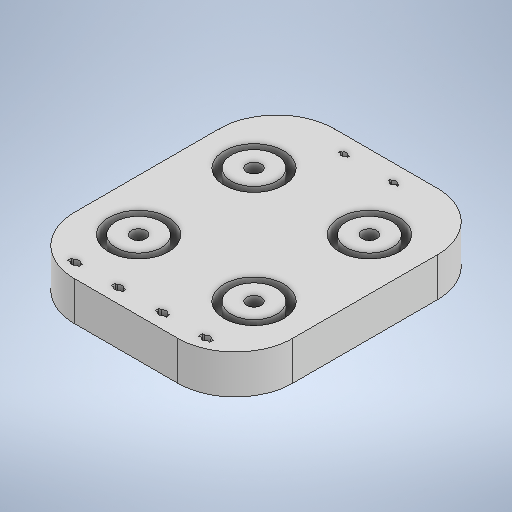
# Autodesk Inventor part: BlenderCase
Saved by Autodesk Inventor 2025 (Build 290162000, 162)
## iProperties
Created: 2025-02-08
Part Number: BlenderCase
Material: Generic
Document SubType Name: Modeling
Designer: ethan
Density: 1 g/cm^3
Appearance: Default
Author: ethan
Autodesk Inventor part; units mm, degrees
ref_plane "YZ Plane" through (0, 0, 0) normal (1, 0, 0) x (0, 1, 0)
ref_plane "XZ Plane" through (0, 0, 0) normal (0, 1, 0) x (-1, 0, 0)
ref_plane "XY Plane" through (0, 0, 0) normal (0, 0, 1) x (1, 0, 0)
sketch "Sketch1" plane through (0, 0, 0) normal (0, 1, 0) x (-1, 0, 0)
  circle A0 centre (0, 0) radius 26.1938
  circle A1 centre (0, 0) radius 19.8438
  circle A2 centre (0, 0) radius 32.5438
  dimension "d0" = 52.3875
  dimension "d1" = 6.35
  dimension "d2" = 6.35
  constraints: 3 centre point, 1 coincident
  measures "d0" diameter of A0
  measures "d1" radial gap between concentric circles of A0 A1
  measures "d2" radial gap between concentric circles of A0 A2
extrude "Extrusion1" add sketch "Sketch1" along normal blind 31.75
sketch "Sketch2" plane through (0, 31.75, 0) normal (0, 1, 0) x (1, 0, 0)
  circle A0 centre (0, 0) radius 6.35
  dimension "d5" = 12.7
  constraints: 1 centre point, 1 coincident
  measures "d5" diameter of A0
extrude "Extrusion2" cut sketch "Sketch2" against normal blind 31.75
sketch "Sketch3" plane through (0, 31.75, 0) normal (0, 1, 0) x (1, 0, 0)
  circle A0 centre (0, 0) radius 32.5438 construction
  circle A1 centre (0, 0) radius 32.5438 construction
  circle A2 centre (0, 0) radius 26.1938 construction
  circle A3 centre (0, 0) radius 26.1938 construction
  circle A4 centre (0, 0) radius 19.8438 construction
  circle A5 centre (0, 0) radius 19.8438 construction
  circle A6 centre (0, 0) radius 6.35 construction
  circle A7 centre (0, 0) radius 6.35 construction
  circle A8 centre (0, 0) radius 32.5438 construction
  circle A9 centre (0, 0) radius 26.1938 construction
  circle A10 centre (0, 0) radius 32.5438 construction
  circle A11 centre (0, 0) radius 26.1938 construction
  circle A12 centre (0, 0) radius 32.5438 construction
  circle A13 centre (0, 0) radius 32.5438 construction
  circle A14 centre (0, 0) radius 26.1938 construction
  circle A15 centre (0, 0) radius 26.1938 construction
  circle A16 centre (0, 0) radius 6.35 construction
  circle A17 centre (0, 0) radius 19.8438 construction
  circle A18 centre (0, 0) radius 6.35 construction
  circle A19 centre (0, 0) radius 19.8438 construction
  circle A20 centre (0, 0) radius 19.8438 construction
  circle A21 centre (0, 0) radius 19.8438 construction
  circle A22 centre (0, 0) radius 6.35 construction
  circle A23 centre (0, 0) radius 6.35 construction
  line L0 (0, 0) -> (101.6, 0) construction
  line L1 (101.6, 0) -> (101.6, -101.6) construction
  circle A24 centre (0, 0) radius 6.35
  circle A25 centre (0, 0) radius 19.8438
  circle A26 centre (0, 0) radius 26.1938
  circle A27 centre (0, 0) radius 32.5438
  circle A28 centre (101.6, 0) radius 19.8438
  circle A29 centre (101.6, 0) radius 26.1938
  circle A30 centre (101.6, 0) radius 6.35
  circle A31 centre (101.6, 0) radius 32.5438
  circle A32 centre (0, -101.6) radius 19.8438
  circle A33 centre (0, -101.6) radius 26.1938
  circle A34 centre (0, -101.6) radius 6.35
  circle A35 centre (0, -101.6) radius 32.5438
  circle A36 centre (101.6, -101.6) radius 19.8438
  circle A37 centre (101.6, -101.6) radius 26.1938
  circle A38 centre (101.6, -101.6) radius 6.35
  circle A39 centre (101.6, -101.6) radius 32.5438
  line L2 (0, 0) -> (50.8, 87.9882) construction
  line L3 (50.8, 87.9882) -> (101.6, 0) construction
  line L4 (16.2719, 28.1837) -> (28.9719, 50.1808) construction
  line L5 (28.9719, 50.1808) -> (72.6281, 50.1808) construction
  circle A40 centre (28.9719, 50.1808) radius 2.3812
  circle A41 centre (72.6281, 50.1808) radius 2.3813
  line L6 (25.0031, 49.387) -> (32.9406, 49.387)
  line L7 (32.9406, 49.387) -> (32.9406, 50.9745)
  line L8 (32.9406, 50.9745) -> (25.0031, 50.9745)
  line L9 (25.0031, 50.9745) -> (25.0031, 49.387)
  line L10 (25.0031, 49.387) -> (32.9406, 50.9745) construction
  line L11 (32.9406, 49.387) -> (25.0031, 50.9745) construction
  line L12 (68.6594, 49.387) -> (76.5969, 49.387)
  line L13 (76.5969, 49.387) -> (76.5969, 50.9745)
  line L14 (76.5969, 50.9745) -> (68.6594, 50.9745)
  line L15 (68.6594, 50.9745) -> (68.6594, 49.387)
  line L16 (68.6594, 49.387) -> (76.5969, 50.9745) construction
  line L17 (76.5969, 49.387) -> (68.6594, 50.9745) construction
  line L18 (28.9719, 52.562) -> (28.9719, 65.262) construction
  line L19 (-107.0093, 65.262) -> (-107.0093, -188.738) construction
  line L20 (-32.5438, -101.6) -> (-45.2437, -101.6) construction
  line L21 (134.1437, -101.6) -> (146.8437, -101.6) construction
  line L22 (-45.2437, -188.738) -> (146.8438, -188.738) construction
  line L23 (-45.2437, -188.738) -> (-45.2437, -163.338) construction
  line L24 (-45.2437, 65.262) -> (96.0437, 65.262) construction
  line L25 (146.8438, 65.262) -> (146.8438, -112.538) construction
  line L26 (96.0437, -163.338) -> (5.5563, -163.338) construction
  line L27 (-45.2437, -112.538) -> (-45.2437, 65.262) construction
  line L28 (-45.2437, -163.338) -> (-6.8237, -163.338) construction
  line L29 (-6.8237, -163.338) -> (-6.8237, -150.638) construction
  line L30 (-6.8237, -163.338) -> (31.5963, -163.338) construction
  line L31 (31.5963, -163.338) -> (70.0164, -163.338) construction
  line L32 (70.0164, -163.338) -> (108.4364, -163.338) construction
  line L33 (108.4364, -163.338) -> (146.8438, -163.338) construction
  circle A42 centre (-6.8237, -150.638) radius 3.175 construction
  circle A43 centre (31.5963, -150.638) radius 3.175 construction
  circle A44 centre (70.0164, -150.638) radius 3.175 construction
  circle A45 centre (108.4364, -150.638) radius 3.175 construction
  circle A46 centre (-6.8237, -150.638) radius 3.175
  circle A47 centre (31.5963, -150.638) radius 3.175
  circle A48 centre (70.0164, -150.638) radius 3.175
  circle A49 centre (108.4364, -150.638) radius 3.175
  line L34 (-11.5862, -152.2255) -> (-2.0612, -152.2255)
  line L35 (-2.0612, -152.2255) -> (-2.0612, -149.0505)
  line L36 (-2.0612, -149.0505) -> (-11.5862, -149.0505)
  line L37 (-11.5862, -149.0505) -> (-11.5862, -152.2255)
  line L38 (-11.5862, -152.2255) -> (-2.0612, -149.0505) construction
  line L39 (-2.0612, -152.2255) -> (-11.5862, -149.0505) construction
  line L40 (26.8338, -152.2255) -> (36.3588, -152.2255)
  line L41 (36.3588, -152.2255) -> (36.3588, -149.0505)
  line L42 (36.3588, -149.0505) -> (26.8338, -149.0505)
  line L43 (26.8338, -149.0505) -> (26.8338, -152.2255)
  line L44 (26.8338, -152.2255) -> (36.3588, -149.0505) construction
  line L45 (36.3588, -152.2255) -> (26.8338, -149.0505) construction
  line L46 (65.2539, -152.2255) -> (74.7789, -152.2255)
  line L47 (74.7789, -152.2255) -> (74.7789, -149.0505)
  line L48 (74.7789, -149.0505) -> (65.2539, -149.0505)
  line L49 (65.2539, -149.0505) -> (65.2539, -152.2255)
  line L50 (65.2539, -152.2255) -> (74.7789, -149.0505) construction
  line L51 (74.7789, -152.2255) -> (65.2539, -149.0505) construction
  line L52 (103.6739, -152.2255) -> (113.1989, -152.2255)
  line L53 (113.1989, -152.2255) -> (113.1989, -149.0505)
  line L54 (113.1989, -149.0505) -> (103.6739, -149.0505)
  line L55 (103.6739, -149.0505) -> (103.6739, -152.2255)
  line L56 (103.6739, -152.2255) -> (113.1989, -149.0505) construction
  line L57 (113.1989, -152.2255) -> (103.6739, -149.0505) construction
  line L58 (-45.2437, -163.338) -> (146.8438, -163.338)
  line L59 (146.8438, -163.338) -> (146.8438, 14.462)
  line L60 (146.8438, 65.262) -> (5.5563, 65.262)
  line L61 (-45.2437, 14.462) -> (-45.2437, -163.338)
  arc A50 (5.5563, 65.262) -> (-45.2437, 14.462) centre (5.5563, 14.462) ccw
  arc A51 (146.8438, 14.462) -> (96.0437, 65.262) centre (96.0438, 14.462) ccw
  arc A52 (96.0437, -163.338) -> (146.8438, -112.538) centre (96.0438, -112.538) ccw
  arc A53 (-45.2437, -112.538) -> (5.5563, -163.338) centre (5.5563, -112.538) ccw
  point P0 (31.2169, 49.387)
  point P1 (26.7268, 49.387)
  point P2 (26.7268, 50.9745)
  point P3 (31.2169, 50.9745)
  point P4 (74.8732, 49.387)
  point P5 (70.3831, 49.387)
  point P6 (70.3831, 50.9745)
  point P7 (74.8732, 50.9745)
  point P8 (-4.0741, -152.2255)
  point P9 (-9.5733, -152.2255)
  point P10 (-9.5733, -149.0505)
  point P11 (-4.0741, -149.0505)
  point P12 (34.346, -152.2255)
  point P13 (28.8467, -152.2255)
  point P14 (28.8467, -149.0505)
  point P15 (34.346, -149.0505)
  point P16 (72.766, -152.2255)
  point P17 (67.2667, -152.2255)
  point P18 (67.2667, -149.0505)
  point P19 (72.766, -149.0505)
  point P20 (111.186, -152.2255)
  point P21 (105.6868, -152.2255)
  point P22 (105.6868, -149.0505)
  point P23 (111.186, -149.0505)
  dimension "d20" = 4.7625
  dimension "d8" = 101.6
  dimension "d9" = 101.6
  dimension "d12" = 101.6
  dimension "d15" = 101.6
  dimension "d18" = 101.6
  dimension "d19" = 25.4
  dimension "d21" = 4.7625
  dimension "d22" = 7.9375
  dimension "d23" = 1.5875
  dimension "d24" = 7.9375
  dimension "d25" = 1.5875
  dimension "d26" = 12.7
  dimension "d27" = 254
  dimension "d28" = 12.7
  dimension "d29" = 12.7
  dimension "d30" = 25.4
  dimension "d31" = 38.42
  dimension "d32" = 12.7
  dimension "d33" = 38.42
  dimension "d34" = 38.42
  dimension "d35" = 38.42
  dimension "d36" = 6.35
  dimension "d37" = 6.35
  dimension "d38" = 6.35
  dimension "d39" = 6.35
  dimension "d40" = 9.525
  dimension "d41" = 3.175
  dimension "d42" = 9.525
  dimension "d43" = 3.175
  dimension "d44" = 9.525
  dimension "d45" = 3.175
  dimension "d46" = 9.525
  dimension "d47" = 3.175
  dimension "d48" = 50.8
  constraints: 124 end point, 26 centre point, 23 coincident, 16 parallel, 13 point on line, 12 midpoint, 11 perpendicular, 10 horizontal, 8 equal radius, 8 point on circle, 8 tangent, 6 vertical, 2 horizontal alignment, 2 line through centre, 1 collinear, 106 other
  measures "d8" distance of L0.start L0.end
  measures "d9" distance of L0.end L1.end
  measures "d12" distance of A25.centre A28.centre
  measures "d15" distance of A25.centre A32.centre
  measures "d18" distance of L2.start L2.end
  measures "d19" distance of L4.start L4.end
  measures "d21" diameter of A41
  measures "d22" distance of L6.start L6.end
  measures "d23" distance of L7.end L6.end
  measures "d24" distance of L12.start L12.end
  measures "d25" distance of L13.end L12.end
  measures "d26" distance of L18.start L18.end
  measures "d27" distance of L19.start L19.end
  measures "d28" distance of L20.start L20.end
  measures "d29" distance of L21.start L21.end
  measures "d30" distance of L22.start L23.end
  measures "d31" distance of L28.start L28.end
  measures "d32" distance of L28.end L29.end
  measures "d33" distance of L28.end L30.end
  measures "d34" distance of L30.end L31.end
  measures "d35" distance of L31.end L32.end
  measures "d36" diameter of A42
  measures "d37" diameter of A43
  measures "d38" diameter of A44
  measures "d39" diameter of A45
  measures "d40" distance of L34.start L34.end
  measures "d41" distance of L35.end L34.end
  measures "d42" distance of L40.start L40.end
  measures "d43" distance of L41.end L40.end
  measures "d44" distance of L46.start L46.end
  measures "d45" distance of L47.end L46.end
  measures "d46" distance of L52.start L52.end
  measures "d47" distance of L53.end L52.end
  measures "d48" radius of A50
extrude "Extrusion3" add sketch "Sketch3" against normal blind 31.75 contours A28 | A31 | A32 | A35 | A36 | A39 | A53 L61 A50 L60 A51 L59 A52 L58
sketch "Sketch4" plane through (0, 0, 0) normal (0, -1, 0) x (1, 0, 0)
  line L0 (113.1989, 152.2255) -> (113.1989, 149.0505) projected
  line L1 (113.1989, 149.0505) -> (111.186, 149.0505) projected
  arc A0 (105.6868, 149.0505) -> (111.186, 149.0505) centre (108.4364, 150.638) ccw projected
  line L2 (105.6868, 149.0505) -> (103.6739, 149.0505) projected
  line L3 (103.6739, 149.0505) -> (103.6739, 152.2255) projected
  line L4 (103.6739, 152.2255) -> (105.6868, 152.2255) projected
  arc A1 (111.186, 152.2255) -> (105.6868, 152.2255) centre (108.4364, 150.638) ccw projected
  line L5 (111.186, 152.2255) -> (113.1989, 152.2255) projected
  line L6 (74.7789, 152.2255) -> (74.7789, 149.0505) projected
  line L7 (74.7789, 149.0505) -> (72.766, 149.0505) projected
  arc A2 (67.2667, 149.0505) -> (72.766, 149.0505) centre (70.0164, 150.638) ccw projected
  line L8 (67.2667, 149.0505) -> (65.2539, 149.0505) projected
  line L9 (65.2539, 149.0505) -> (65.2539, 152.2255) projected
  line L10 (65.2539, 152.2255) -> (67.2667, 152.2255) projected
  arc A3 (72.766, 152.2255) -> (67.2667, 152.2255) centre (70.0164, 150.638) ccw projected
  line L11 (72.766, 152.2255) -> (74.7789, 152.2255) projected
  line L12 (36.3588, 152.2255) -> (36.3588, 149.0505) projected
  line L13 (36.3588, 149.0505) -> (34.346, 149.0505) projected
  arc A4 (28.8467, 149.0505) -> (34.346, 149.0505) centre (31.5963, 150.638) ccw projected
  line L14 (28.8467, 149.0505) -> (26.8338, 149.0505) projected
  line L15 (26.8338, 149.0505) -> (26.8338, 152.2255) projected
  line L16 (26.8338, 152.2255) -> (28.8467, 152.2255) projected
  arc A5 (34.346, 152.2255) -> (28.8467, 152.2255) centre (31.5963, 150.638) ccw projected
  line L17 (34.346, 152.2255) -> (36.3588, 152.2255) projected
  line L18 (-2.0612, 152.2255) -> (-2.0612, 149.0505) projected
  line L19 (-2.0612, 149.0505) -> (-4.0741, 149.0505) projected
  arc A6 (-9.5733, 149.0505) -> (-4.0741, 149.0505) centre (-6.8237, 150.638) ccw projected
  line L20 (-9.5733, 149.0505) -> (-11.5862, 149.0505) projected
  line L21 (-11.5862, 149.0505) -> (-11.5862, 152.2255) projected
  line L22 (-11.5862, 152.2255) -> (-9.5733, 152.2255) projected
  arc A7 (-4.0741, 152.2255) -> (-9.5733, 152.2255) centre (-6.8237, 150.638) ccw projected
  line L23 (-4.0741, 152.2255) -> (-2.0612, 152.2255) projected
  line L24 (76.5969, -49.387) -> (76.5969, -50.9745) projected
  line L25 (76.5969, -50.9745) -> (74.8732, -50.9745) projected
  arc A8 (70.3831, -50.9745) -> (74.8732, -50.9745) centre (72.6281, -50.1808) ccw projected
  line L26 (70.3831, -50.9745) -> (68.6594, -50.9745) projected
  line L27 (68.6594, -50.9745) -> (68.6594, -49.387) projected
  line L28 (68.6594, -49.387) -> (70.3831, -49.387) projected
  arc A9 (74.8732, -49.387) -> (70.3831, -49.387) centre (72.6281, -50.1808) ccw projected
  line L29 (74.8732, -49.387) -> (76.5969, -49.387) projected
  line L30 (32.9406, -49.387) -> (32.9406, -50.9745) projected
  line L31 (32.9406, -50.9745) -> (31.2169, -50.9745) projected
  arc A10 (26.7268, -50.9745) -> (31.2169, -50.9745) centre (28.9719, -50.1808) ccw projected
  line L32 (26.7268, -50.9745) -> (25.0031, -50.9745) projected
  line L33 (25.0031, -50.9745) -> (25.0031, -49.387) projected
  line L34 (25.0031, -49.387) -> (26.7268, -49.387) projected
  arc A11 (31.2169, -49.387) -> (26.7268, -49.387) centre (28.9719, -50.1808) ccw projected
  line L35 (31.2169, -49.387) -> (32.9406, -49.387) projected
  circle A12 centre (101.6, 101.6) radius 26.1938 projected
  circle A13 centre (0, 101.6) radius 26.1938 projected
  circle A14 centre (101.6, 0) radius 26.1938 projected
  line L36 (-45.2437, 112.538) -> (-45.2437, -14.462) projected
  arc A15 (-45.2437, -14.462) -> (5.5563, -65.262) centre (5.5563, -14.462) ccw projected
  line L37 (5.5563, -65.262) -> (96.0437, -65.262) projected
  arc A16 (96.0437, -65.262) -> (146.8438, -14.462) centre (96.0438, -14.462) ccw projected
  line L38 (146.8438, -14.462) -> (146.8438, 112.538) projected
  arc A17 (146.8438, 112.538) -> (96.0437, 163.338) centre (96.0438, 112.538) ccw projected
  line L39 (96.0437, 163.338) -> (5.5563, 163.338) projected
  arc A18 (5.5563, 163.338) -> (-45.2437, 112.538) centre (5.5563, 112.538) ccw projected
  circle A19 centre (0, 0) radius 26.1938 projected
extrude "Extrusion4" add sketch "Sketch4" along normal blind 2.54 contours L0 L1 A0 L2 L3 L4 A1 L5 | L6 L7 A2 L8 L9 L10 A3 L11 | L12 L13 A4 L14 L15 L16 A5 L17 | L18 L19 A6 L20 L21 L22 A7 L23 | L24 L25 A8 L26 L27 L28 A9 L29 | L30 L31 A10 L32 L33 L34 A11 L35 | A12 | A13 | A14 | A18 L39 A17 L38 A16 L37 A15 L36 | A19
shell "Shell1" thickness 2.54 removed faces 1 at (18.7854, -2.54, 27.8713)
body "Solid1"
